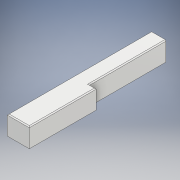
# Autodesk Inventor part: key1
Saved by Autodesk Inventor 2017 (Build 210142000, 142)
## iProperties
Created: 2018-03-15
Part Number: key1
Material: Generic
Document SubType Name: Modeling
Designer: Luiz Gustavo
Density: 1 g/cm^3
Appearance: White
key_width: 23,000 mm
key_length: 150,000 mm
blackkey_length: 80,000 mm
key_height: 20,000 mm
d5: 0,00 deg
blackkey_halfwidth: 7,000 mm
Author: Luiz Gustavo
Autodesk Inventor part; units mm, degrees
ref_plane "YZ Plane" through (0, 0, 0) normal (1, 0, 0) x (0, 1, 0)
ref_plane "XZ Plane" through (0, 0, 0) normal (0, 1, 0) x (-1, 0, 0)
ref_plane "XY Plane" through (0, 0, 0) normal (0, 0, 1) x (1, 0, 0)
sketch "Sketch1" plane through (0, 0, 0) normal (0, 0, 1) x (1, 0, 0)
  line L0 (-11.5, -75) -> (11.5, -75)
  line L1 (11.5, -75) -> (11.5, 75)
  line L2 (11.5, 75) -> (-11.5, 75)
  line L3 (-11.5, 75) -> (-11.5, -75)
  line L4 (-11.5, -75) -> (11.5, 75) construction
  line L5 (11.5, -75) -> (-11.5, 75) construction
  line L6 (11.5, 75) -> (4.5, 75)
  line L7 (4.5, 75) -> (4.5, -5)
  line L8 (4.5, -5) -> (11.5, -5)
  line L9 (11.5, -5) -> (11.5, 75)
  point P0 (0, 0)
  dimension "key_width" = 23
  dimension "key_length" = 150
  dimension "blackkey_length" = 80
  dimension "blackkey_halfwidth" = 7
  constraints: 20 end point, 4 parallel, 2 horizontal, 2 midpoint, 2 perpendicular
  measures "key_width" distance of L0.start L0.end
  measures "key_length" distance of L0.end L1.end
  measures "blackkey_length" distance between parallel lines of L8 L2
  measures "blackkey_halfwidth" distance between parallel lines of L7 L1
extrude "Extrusion1" add sketch "Sketch1" against normal blind 20 contours L3 L2 L7 L8 L1 L0
chamfer "Chamfer1" distance 1 angle 45 5 edges at (11.5, -40, 0) (0, -75, 0) (-11.5, 0, 0) (4.5, 35, 0) (8, -5, 0)
body "Solid1"
